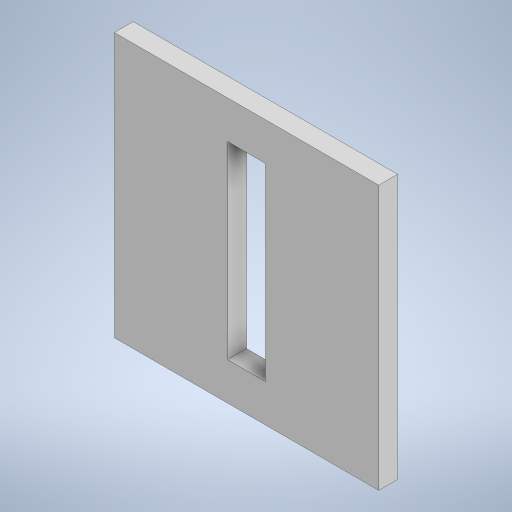
# Autodesk Inventor part: JukeBox Top Panel
Saved by Autodesk Inventor 2024 (Build 280153000, 153)
## iProperties
Created: 2023-04-22
Part Number: JukeBox Top Panel
Material: Generic
Document SubType Name: Modeling
Designer: newic
Density: 1 g/cm^3
Appearance: Default
Author: newic
Autodesk Inventor part; units mm, degrees
ref_plane "YZ Plane" through (0, 0, 0) normal (1, 0, 0) x (0, 1, 0)
ref_plane "XZ Plane" through (0, 0, 0) normal (0, 1, 0) x (-1, 0, 0)
ref_plane "XY Plane" through (0, 0, 0) normal (0, 0, 1) x (1, 0, 0)
sketch "Sketch1" plane through (0, 0, 0) normal (0, 0, 1) x (1, 0, 0)
  line L0 (0, 0) -> (812.8, 0) construction
  line L1 (812.8, 0) -> (812.8, -406.4) construction
  line L2 (812.8, -406.4) -> (0, -406.4) construction
  line L3 (0, -406.4) -> (0, 0) construction
  line L4 (0, 0) -> (406.4, 0)
  line L5 (406.4, 0) -> (406.4, -25.4)
  line L6 (406.4, -25.4) -> (0, -25.4)
  line L7 (0, -25.4) -> (0, 0)
  line L8 (406.4, -25.4) -> (381, -25.4)
  line L9 (381, -25.4) -> (381, -406.4)
  line L10 (381, -406.4) -> (406.4, -406.4)
  line L11 (406.4, -406.4) -> (406.4, -25.4)
  line L12 (381, -406.4) -> (0, -406.4)
  line L13 (0, -406.4) -> (0, -381)
  line L14 (0, -381) -> (381, -381)
  line L15 (381, -381) -> (381, -406.4)
  line L16 (0, -381) -> (25.4, -381)
  line L17 (25.4, -381) -> (25.4, -25.4)
  line L18 (25.4, -25.4) -> (0, -25.4)
  line L19 (0, -25.4) -> (0, -381)
  dimension "d1" = 812.8
  dimension "d5" = 406.4
  dimension "d6" = 25.4
  dimension "d7" = 25.4
  dimension "d8" = 381
  dimension "d9" = 381
  dimension "d10" = 25.4
  dimension "d11" = 25.4
  constraints: 32 end point, 8 parallel, 4 horizontal, 4 perpendicular, 1 point on line, 2 other
  measures "d1" distance of L1.end L2.end
  measures "d5" distance of L5.end L6.end
  measures "d6" distance of L4.end L5.end
  measures "d7" distance of L10.end L9.end
  measures "d8" distance of L9.end L8.end
  measures "d9" distance of L13.end L14.end
  measures "d10" distance of L12.end L13.end
  measures "d11" distance of L18.end L17.end
extrude "Extrusion1" add sketch "Sketch1" against normal blind 25.4 contours L6 L9 L14 L17
sketch "Sketch2" plane through (0, 0, 0) normal (0, 0, 1) x (1, 0, 0)
  line L0 (0, 0) -> (812.8, 0) construction
  line L1 (812.8, 0) -> (812.8, -406.4) construction
  line L2 (812.8, -406.4) -> (0, -406.4) construction
  line L3 (0, -406.4) -> (0, 0) construction
  line L4 (406.4, 0) -> (228.6, 0)
  line L5 (228.6, 0) -> (228.6, -76.2)
  line L6 (228.6, -76.2) -> (406.4, -76.2)
  line L7 (406.4, -76.2) -> (406.4, 0)
  line L8 (228.6, -76.2) -> (177.8, -76.2)
  line L9 (177.8, -76.2) -> (177.8, -330.2)
  line L10 (177.8, -330.2) -> (228.6, -330.2)
  line L11 (228.6, -330.2) -> (228.6, -76.2)
  dimension "d15" = 812.8
  dimension "d27" = 177.8
  dimension "d28" = 76.2
  dimension "d30" = 50.8
  dimension "d31" = 254
  constraints: 16 end point, 4 parallel, 2 horizontal, 2 perpendicular, 1 midpoint, 2 other
  measures "d15" distance of L1.end L2.end
  measures "d27" distance of L6.end L5.end
  measures "d28" distance of L5.end L4.end
  measures "d30" distance of L10.end L9.end
  measures "d31" distance of L9.end L8.end
extrude "Extrusion2" cut sketch "Sketch2" against normal blind 25.4 contours L11 L10 L9 L8
body "Solid1"
